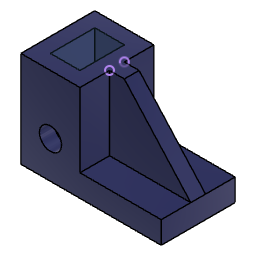
Exercise 3_ (Autodesk Fusion 360 design; units mm, degrees)
Autodesk Fusion 360 part; units mm, degrees
sketch "Sketch1" plane through (0, 0, 0) normal (0, 1, 0) x (1, 0, 0)
  line L0 (0, 0) -> (95, 0)
  line L1 (95, 0) -> (95, -15)
  line L2 (95, -15) -> (40, -15)
  line L3 (40, -15) -> (40, -65)
  line L4 (40, -65) -> (0, -65)
  line L5 (0, -65) -> (0, 0)
  dimension "d1" = 95
  constraint coincident L0.start L5.end
  constraint horizontal L0
  constraint perpendicular L0 L1
  constraint perpendicular L1 L2
  constraint perpendicular L2 L3
  constraint perpendicular L3 L4
  constraint perpendicular L0 L5
  measures "d1" distance of L0.start L0.end
extrude "Extrude1" add sketch "Sketch1" along normal blind 50
sketch "Sketch2" plane through (0, 0, 65) normal (0, 0, 1) x (-1, 0, 0)
  line L0 (0, 0) -> (-40, 0)
  line L1 (-40, 0) -> (-40, -50)
  line L2 (-40, -50) -> (0, -50)
  line L3 (0, -50) -> (0, 0)
  line L4 (7.2091, -40) -> (5, -40)
  line L5 (-10, -10) -> (-30, -10)
  line L6 (-10, -40) -> (-30, -40)
  line L7 (-30, -10) -> (-30, -40)
  line L8 (-10, -10) -> (-10, -40)
  constraint perpendicular L3 L4
extrude "Extrude2" cut sketch "Sketch2" against normal blind 90 contours L5 L6 L7 L8
sketch "Sketch3" plane through (0, 0, 0) normal (0, -1, 0) x (1, 0, 0)
  line L0 (40, 65) -> (0, 65)
  line L1 (0, 65) -> (0, 0)
  line L2 (0, 0) -> (95, 0)
  line L3 (95, 0) -> (95, 15)
  line L4 (95, 15) -> (40, 15)
  line L5 (40, 15) -> (40, 65)
  line L6 (-20, 25) -> (0, 25)
  circle A0 centre (20, 25) radius 7.5
  line L7 (20, 0) -> (20, -6.3794)
  dimension "d15" = 25
  dimension "d16" = 15
  constraint horizontal L6
  constraint coincident L1 L6.end
  constraint coincident L2 L7.start
  measures "d15" distance of L2 L6
  measures "d16" diameter of A0
extrude "Extrude3" cut sketch "Sketch3" against normal blind 20 contours A0
sketch "Sketch4" plane through (0, 0, 15) normal (0, 0, 1) x (-1, 0, 0)
  line L0 (-40, 0) -> (-95, 0)
  line L1 (-95, 0) -> (-95, -50)
  line L2 (-95, -50) -> (-40, -50)
  line L3 (-40, -50) -> (-40, 0)
  line L4 (-40, -20) -> (-95, -20)
  line L5 (-40, -30) -> (-95, -30)
  constraint coincident L3 L4.start
  constraint perpendicular L3 L4
  constraint coincident L3 L5.start
  constraint perpendicular L1 L5
  constraint coincident L1 L4.end
  constraint coincident L1 L5.end
extrude "Extrude4" add sketch "Sketch4" along normal blind 50 contours L1 L3 L4 L5
sketch "Sketch5" plane through (0, 0, 65) normal (0, 0, 1) x (-1, 0, 0)
  line L0 (-10, -40) -> (-30, -40)
  line L1 (-30, -40) -> (-30, -10)
  line L2 (-30, -10) -> (-10, -10)
  line L3 (-10, -10) -> (-10, -40)
  line L4 (0, 0) -> (-40, 0)
  line L5 (-40, 0) -> (-40, -20)
  line L6 (-40, -30) -> (-40, -50)
  line L7 (-40, -50) -> (0, -50)
  line L8 (0, -50) -> (0, 0)
sketch "Sketch6" plane through (0, 20, 0) normal (0, -1, 0) x (1, 0, 0)
  line L0 (40, 15) -> (95, 15)
  line L1 (95, 15) -> (95, 65)
  line L2 (95, 65) -> (40, 65)
  line L3 (40, 65) -> (40, 15)
  line L4 (50, 65) -> (95, 15)
  point P0 (50, 65)
  constraint coincident P0 L4.start
  constraint coincident L0.end L1.start
extrude "Extrude5" cut sketch "Sketch6" against normal blind 65 contours L1 L2 L4
sketch "Sketch7" plane through (0, 0, 0) normal (0, 1, 0) x (1, 0, 0)
